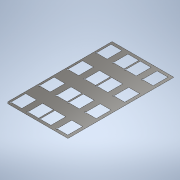
# Autodesk Inventor part: Assembly Stencil
Saved by Autodesk Inventor 2022 (Build 260153000, 153)
## iProperties
Created: 2021-01-11
Part Number: Assembly Stencil
Material: Stainless Steel
Document SubType Name: Modeling
Designer: caleb
Density: 8 g/cm^3
Appearance: Semi-Polished
Author: caleb
Autodesk Inventor part; units mm, degrees
ref_plane "YZ Plane" through (0, 0, 0) normal (1, 0, 0) x (0, 1, 0)
ref_plane "XZ Plane" through (0, 0, 0) normal (0, 1, 0) x (-1, 0, 0)
ref_plane "XY Plane" through (0, 0, 0) normal (0, 0, 1) x (1, 0, 0)
sketch "Sketch1" plane through (0, 0, 0) normal (0, 1, 0) x (-1, 0, 0)
  line L0 (-62.23, 106.68) -> (62.23, 106.68)
  line L1 (62.23, 106.68) -> (62.23, -106.68)
  line L2 (62.23, -106.68) -> (-62.23, -106.68)
  line L3 (-62.23, -106.68) -> (-62.23, 106.68)
  line L4 (-62.23, 106.68) -> (62.23, -106.68) construction
  line L5 (62.23, 106.68) -> (-62.23, -106.68) construction
  point P0 (0, 0)
  dimension "d0" = 213.36
  dimension "d1" = 124.46
  constraints: 12 end point, 2 midpoint, 2 parallel, 1 horizontal, 1 perpendicular
  measures "d0" distance of L0.end L1.end
  measures "d1" distance of L0.start L0.end
extrude "Extrusion1" add sketch "Sketch1" along normal blind 0.1
chamfer "Chamfer1" distance 3.175 angle 45 1 edges at (-62.23, 0.05, 106.68)
sketch "Sketch2" plane through (0, 0.1, 0) normal (0, 1, 0) x (1, 0, 0)
  line L0 (-36.5, -100.95) -> (-36.5, -70.95)
  line L1 (-36.5, -70.95) -> (-58.5, -70.95)
  line L2 (-62.23, 106.68) -> (-62.23, -106.68) projected
  line L3 (-62.23, -106.68) -> (62.23, -106.68) projected
  arc A0 (-58.5, -99.45) -> (-57, -100.95) centre (-58.5, -100.95) ccw
  line L4 (-36.5, -100.95) -> (-57, -100.95)
  line L5 (-58.5, -99.45) -> (-58.5, -70.95)
  line L6 (56.23, -70.95) -> (34.23, -70.95)
  line L7 (34.23, -70.95) -> (34.23, -99.45)
  line L8 (56.23, -70.95) -> (56.23, -100.95)
  line L9 (62.23, -106.68) -> (62.23, 106.68) projected
  line L10 (35.73, -100.95) -> (56.23, -100.95)
  line L11 (-36.5, -43.633) -> (-36.5, -13.633)
  line L12 (-36.5, -43.633) -> (-57, -43.633)
  line L13 (-36.5, -13.633) -> (-58.5, -13.633)
  line L14 (-58.5, -42.133) -> (-58.5, -13.633)
  arc A1 (-58.5, -42.133) -> (-57, -43.633) centre (-58.5, -43.633) ccw
  line L15 (-36.5, 13.684) -> (-36.5, 43.684)
  line L16 (-36.5, 13.684) -> (-57, 13.684)
  line L17 (-36.5, 43.684) -> (-58.5, 43.684)
  line L18 (-58.5, 15.184) -> (-58.5, 43.684)
  arc A2 (-58.5, 15.184) -> (-57, 13.684) centre (-58.5, 13.684) ccw
  line L19 (-36.5, 71.001) -> (-36.5, 101.001)
  line L20 (-36.5, 71.001) -> (-57, 71.001)
  line L21 (-36.5, 101.001) -> (-58.5, 101.001)
  line L22 (-58.5, 72.501) -> (-58.5, 101.001)
  arc A3 (-58.5, 72.501) -> (-57, 71.001) centre (-58.5, 71.001) ccw
  line L23 (-2.5, -100.95) -> (-2.5, -70.95)
  line L24 (-2.5, -100.95) -> (-23, -100.95)
  line L25 (-2.5, -70.95) -> (-24.5, -70.95)
  line L26 (-24.5, -99.45) -> (-24.5, -70.95)
  arc A4 (-24.5, -99.45) -> (-23, -100.95) centre (-24.5, -100.95) ccw
  line L27 (-2.5, -43.633) -> (-2.5, -13.633)
  line L28 (-2.5, -43.633) -> (-23, -43.633)
  line L29 (-2.5, -13.633) -> (-24.5, -13.633)
  line L30 (-24.5, -42.133) -> (-24.5, -13.633)
  arc A5 (-24.5, -42.133) -> (-23, -43.633) centre (-24.5, -43.633) ccw
  line L31 (-2.5, 13.684) -> (-2.5, 43.684)
  line L32 (-2.5, 13.684) -> (-23, 13.684)
  line L33 (-2.5, 43.684) -> (-24.5, 43.684)
  line L34 (-24.5, 15.184) -> (-24.5, 43.684)
  arc A6 (-24.5, 15.184) -> (-23, 13.684) centre (-24.5, 13.684) ccw
  line L35 (-2.5, 71.001) -> (-2.5, 101.001)
  line L36 (-2.5, 71.001) -> (-23, 71.001)
  line L37 (-2.5, 101.001) -> (-24.5, 101.001)
  line L38 (-24.5, 72.501) -> (-24.5, 101.001)
  arc A7 (-24.5, 72.501) -> (-23, 71.001) centre (-24.5, 71.001) ccw
  arc A8 (34.23, -99.45) -> (35.73, -100.95) centre (34.23, -100.95) ccw
  arc A9 (34.23, -42.133) -> (35.73, -43.633) centre (34.23, -43.633) ccw
  line L39 (34.23, -13.633) -> (34.23, -42.133)
  line L40 (56.23, -13.633) -> (34.23, -13.633)
  line L41 (35.73, -43.633) -> (56.23, -43.633)
  line L42 (56.23, -13.633) -> (56.23, -43.633)
  arc A10 (34.23, 15.184) -> (35.73, 13.684) centre (34.23, 13.684) ccw
  line L43 (34.23, 43.684) -> (34.23, 15.184)
  line L44 (56.23, 43.684) -> (34.23, 43.684)
  line L45 (35.73, 13.684) -> (56.23, 13.684)
  line L46 (56.23, 43.684) -> (56.23, 13.684)
  arc A11 (34.23, 72.501) -> (35.73, 71.001) centre (34.23, 71.001) ccw
  line L47 (34.23, 101.001) -> (34.23, 72.501)
  line L48 (56.23, 101.001) -> (34.23, 101.001)
  line L49 (35.73, 71.001) -> (56.23, 71.001)
  line L50 (56.23, 101.001) -> (56.23, 71.001)
  arc A12 (0.23, -99.45) -> (1.73, -100.95) centre (0.23, -100.95) ccw
  line L51 (0.23, -70.95) -> (0.23, -99.45)
  line L52 (22.23, -70.95) -> (0.23, -70.95)
  line L53 (1.73, -100.95) -> (22.23, -100.95)
  line L54 (22.23, -70.95) -> (22.23, -100.95)
  arc A13 (0.23, -42.133) -> (1.73, -43.633) centre (0.23, -43.633) ccw
  line L55 (0.23, -13.633) -> (0.23, -42.133)
  line L56 (22.23, -13.633) -> (0.23, -13.633)
  line L57 (1.73, -43.633) -> (22.23, -43.633)
  line L58 (22.23, -13.633) -> (22.23, -43.633)
  arc A14 (0.23, 15.184) -> (1.73, 13.684) centre (0.23, 13.684) ccw
  line L59 (0.23, 43.684) -> (0.23, 15.184)
  line L60 (22.23, 43.684) -> (0.23, 43.684)
  line L61 (1.73, 13.684) -> (22.23, 13.684)
  line L62 (22.23, 43.684) -> (22.23, 13.684)
  arc A15 (0.23, 72.501) -> (1.73, 71.001) centre (0.23, 71.001) ccw
  line L63 (0.23, 101.001) -> (0.23, 72.501)
  line L64 (22.23, 101.001) -> (0.23, 101.001)
  line L65 (1.73, 71.001) -> (22.23, 71.001)
  line L66 (22.23, 101.001) -> (22.23, 71.001)
  dimension "d46" = 1.5
  dimension "d47" = 30
  dimension "d50" = 5.73
  dimension "d51" = 3.73
  dimension "d56" = 6
  dimension "d59" = 5.73
  dimension "d62" = 57.317
  dimension "d65" = 34
  dimension "d77" = 22
  dimension "d78" = 22
  dimension "d79" = 1.5
  dimension "d80" = 30
  dimension "d83" = 57.317
  dimension "d86" = 34
  constraints: 128 end point, 32 point on circle, 16 centre point, 4 horizontal, 4 vertical, 2 collinear, 2 horizontal alignment, 2 perpendicular, 2 vertical alignment, 1 parallel, 152 other
  measures "d46" radius of A0
  measures "d47" distance of L1.end A0.centre
  measures "d50" distance between parallel lines of L3 L4
  measures "d51" distance between parallel lines of L2 L5
  measures "d56" distance between parallel lines of L9 L8
  measures "d59" distance between parallel lines of L3 L10
  measures "d62" distance of L0.end L11.end
  measures "d65" distance of L0.end L23.end
  measures "d77" distance between parallel lines of L0 L5
  measures "d78" distance between parallel lines of L7 L8
  measures "d79" radius of A8
  measures "d80" distance of L6.start L8.end
  measures "d83" distance of L7.end L39.end
  measures "d86" distance of L7.end L51.end
extrude "Extrusion2" cut sketch "Sketch2" against normal through all
fillet "Fillet1" radius 1 5 edges at (62.23, 0.05, 106.68) (-59.055, 0.05, 106.68) (-62.23, 0.05, 103.505) (62.23, 0.05, -106.68) (-62.23, 0.05, -106.68)
equation "\"d59\" = d50"
equation "\"d78\" = d77"
equation "\"d80\" = d47"
body "Solid1"
